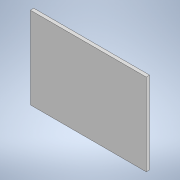
# Autodesk Inventor part: Semrock FF560-Di01-25x36 dichroic beamsplitter
Saved by Autodesk Inventor 2022 (Build 260153000, 153)
## iProperties
Created: 2022-05-01
Part Number: Semrock FF560-Di01-25x36 dichroic beamsplitter
Material: Generic
Document SubType Name: Modeling
Designer: kk4764
Density: 1 g/cm^3
Appearance: Default
Author: kk4764
Autodesk Inventor part; units mm, degrees
ref_plane "YZ Plane" through (0, 0, 0) normal (1, 0, 0) x (0, 1, 0)
ref_plane "XZ Plane" through (0, 0, 0) normal (0, 1, 0) x (-1, 0, 0)
ref_plane "XY Plane" through (0, 0, 0) normal (0, 0, 1) x (1, 0, 0)
sketch "Sketch1" plane through (0, 0, 0) normal (0, 0, 1) x (1, 0, 0)
  line L0 (0, 0) -> (35.6, 0)
  line L1 (35.6, 0) -> (35.6, -25.2)
  line L2 (35.6, -25.2) -> (0, -25.2)
  line L3 (0, -25.2) -> (0, 0)
  dimension "d0" = 25.2
  dimension "d1" = 35.6
  constraints: 8 end point, 2 parallel, 1 horizontal, 1 perpendicular
  measures "d0" distance of L0.end L1.end
  measures "d1" distance of L1.end L2.end
extrude "Extrusion1" add sketch "Sketch1" along normal blind 1.05
body "Solid1"
